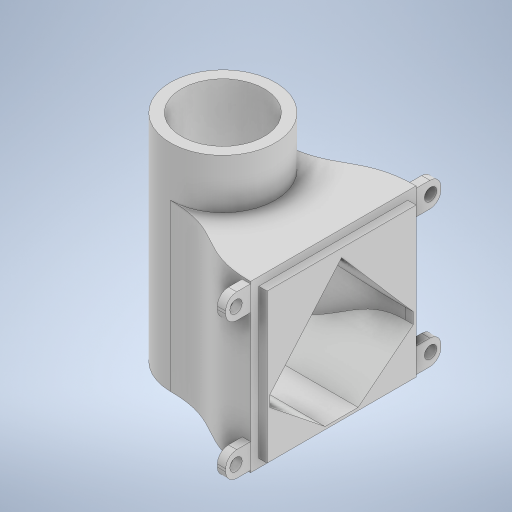
# Autodesk Inventor part: CO-1-01-eStopMountBottom
Saved by Autodesk Inventor 2024 (Build 280153000, 153)
## iProperties
Created: 2023-11-21
Part Number: CO-1-01-eStopMountBottom
Material: Generic
Document SubType Name: Modeling
Designer: t205b
Density: 1 g/cm^3
Appearance: Default
Author: t205b
Autodesk Inventor part; units mm, degrees
ref_plane "XZ Plane" through (0, 0, 0) normal (0, 1, 0) x (-1, 0, 0)
ref_plane "XY Plane" through (0, 0, 0) normal (0, 0, 1) x (1, 0, 0)
sketch "Sketch1" plane through (0, 0, 0) normal (0, 1, 0) x (-1, 0, 0)
  circle A0 centre (0, 0) radius 7.5
  circle A1 centre (0, 0) radius 9.5
  dimension "d0" = 19
  dimension "d1" = 2
  constraints: 2 centre point, 2 coincident
  measures "d0" diameter of A1
  measures "d1" radial gap between concentric circles of A0 A1
extrude "Extrusion1" add sketch "Sketch1" along normal blind 12
ref_plane "Work Plane1" through (9.5, 0, 0) normal (1, 0, 0) x (0, 1, 0)
sketch "Sketch2" plane through (9.5, 0, 0) normal (1, 0, 0) x (0, 1, 0)
  line L0 (-27, 15) -> (-27, -15)
  line L1 (-27, -15) -> (3, -15)
  line L2 (3, -15) -> (3, 15)
  line L3 (3, 15) -> (-27, 15)
  line L4 (-17, -13) -> (-15, -13)
  line L5 (-15, -13) -> (0, 0)
  line L6 (0, 0) -> (-15, 13)
  line L7 (-15, 13) -> (-17, 13)
  line L8 (0, 9.5) -> (12, 9.5) projected
  line L9 (0, -9.5) -> (12, -9.5) projected
  line L10 (0, -9.5) -> (0, 9.5) projected
  line L11 (-25, 3) -> (-25, -3)
  line L12 (-25, -3) -> (-17, -13)
  line L13 (-25, 3) -> (-17, 13)
  line L14 (-22.8, 0) -> (17.8, 0) projected
  line L15 (3, -10.2382) -> (-1.1045, -15)
  point P0 (0, 0)
  dimension "d5" = 30
  dimension "d6" = 2
  dimension "d7" = 2
  dimension "d9" = 26
  dimension "d10" = 13
  dimension "d11" = 3
  dimension "d12" = 3
  dimension "d13" = 30
  dimension "d17" = 2
  dimension "d18" = 2
  dimension "d20" = 2
  dimension "d21" = 6
  dimension "d22" = 3
  dimension "d53" = 15
  dimension "d97" = 8
  dimension "d98" = 8
  constraints: 24 end point, 2 perpendicular, 2 point on line, 2 vertical, 1 parallel
  measures "d5" distance between parallel lines of L1 L3
  measures "d6" distance between parallel lines of L3 L7
  measures "d7" distance between parallel lines of L1 L4
  measures "d9" distance between parallel lines of L7 L4
  measures "d10" distance from line of L5.end L4
  measures "d11" distance from line of L2 L5.end
  measures "d12" distance between parallel lines of L2 L10
  measures "d13" distance of L0.end L1.end
  measures "d17" distance of L4.start L4.end
  measures "d18" distance of L6.end L7.end
  measures "d20" distance between parallel lines of L11 L0
  measures "d21" distance of L11.start L11.end
  measures "d22" distance from line of L14 L11.end
  measures "d53" distance between parallel lines of L14 L1
  measures "d97" horizontal distance of L11.end L4.start
  measures "d98" horizontal distance of L11.start L7.end
extrude "Extrusion2" add sketch "Sketch2" along normal blind 12 and the other way blind 19
sketch "Sketch4" plane through (21.5, 0, 0) normal (1, 0, 0) x (0, 0, -1)
  circle A0 centre (-17.625, -24.375) radius 1.125
  circle A1 centre (-17.625, 0.375) radius 1.125
  circle A2 centre (17.625, -24.375) radius 1.125
  line L0 (7.5, 12) -> (7.5, 3) projected
  circle A3 centre (17.625, 0.375) radius 1.125
  line L1 (-15, 3) -> (-15, -27) projected
  line L2 (-15, -27) -> (15, -27) projected
  line L3 (15, -27) -> (15, 3) projected
  line L4 (15, 3) -> (-15, 3) projected
  line L5 (0, 0) -> (13, -15) projected
  line L6 (13, -15) -> (13, -17) projected
  line L7 (13, -17) -> (3, -25) projected
  line L8 (3, -25) -> (-3, -25) projected
  line L9 (-3, -25) -> (-13, -17) projected
  line L10 (-13, -17) -> (-13, -15) projected
  line L11 (-13, -15) -> (0, 0) projected
  line L12 (-13.5, -25.5) -> (-13.5, 1.5)
  line L13 (-13.5, 1.5) -> (13.5, 1.5)
  line L14 (13.5, 1.5) -> (13.5, -25.5)
  line L15 (13.5, -25.5) -> (-13.5, -25.5)
  point P0 (0, 0)
  dimension "d25" = 2.25
  dimension "d26" = 30
  dimension "d27" = 30
  dimension "d35" = 1.5
  dimension "d55" = 2.625
  dimension "d57" = 2.625
  dimension "d58" = 2.625
  dimension "d61" = 2.625
  dimension "d76" = 2.625
  dimension "d77" = 2.625
  dimension "d78" = 2.625
  dimension "d79" = 2.625
  constraints: 8 end point, 4 centre point, 3 equal radius, 3 other
  measures "d25" diameter of A0
  measures "d26" distance between parallel lines of L3 L1
  measures "d27" distance of L1.start L1.end
  measures "d35" distance between parallel lines of L1 L12
  measures "d55" distance from line of L4 A3.centre
  measures "d57" distance from line of L4 A1.centre
  measures "d58" distance from line of L2 A0.centre
  measures "d61" distance from line of L2 A2.centre
  measures "d76" distance from line of L3 A3.centre
  measures "d77" distance from line of L3 A2.centre
  measures "d78" distance from line of L1 A0.centre
  measures "d79" distance from line of L1 A1.centre
extrude "Extrusion4" cut sketch "Sketch4" against normal blind 1.5 contours L4 L3 L2 L1
sketch "Sketch8" plane through (0, 3, 0) normal (0, 1, 0) x (1, 0, 0)
  point P0 (0, 0)
  point P1 (0, 0)
  constraints: 1 coincident
hole "Hole2" at (0, 3, 0) direction (0, -1, 0) diameter 15 depth 10 tip angle 118
sketch "Sketch9" plane through (0, 3, 0) normal (0, 1, 0) x (1, 0, 0)
  line L0 (20, -15) -> (20, 15) projected
  line L1 (-9.5, 15) -> (20, 15) projected
  line L2 (-9.5, 0) -> (-9.5, 15) projected
  circle A0 centre (0, 0) radius 9.5 projected
  line L3 (-9.5, -15) -> (-9.5, 0) projected
  line L4 (20, -15) -> (-9.5, -15) projected
  line L5 (-9.5, 15) -> (20, 15) projected
  line L6 (0, 9.5) -> (10, 9.5) construction
  line L7 (10, 9.5) -> (10, 15) construction
  line L8 (10, 15) -> (20, 15) construction
  spline S0 degree 3 poles (0, 9.5) (10, 9.5) (10, 15) (20, 15) knots 1 1 1 1 2 2 2 2
  circle A1 centre (0, 0) radius 9.5 projected
  line L9 (-9.5, 15) -> (20, 15) projected
  line L10 (-15.7, 0) -> (27.7, 0) projected
  line L11 (0, -9.5) -> (10, -9.5) construction
  line L12 (10, -9.5) -> (10, -15) construction
  line L13 (10, -15) -> (20, -15) construction
  spline S1 degree 3 poles (0, -9.5) (10, -9.5) (10, -15) (20, -15) knots 1 1 1 1 2 2 2 2
  line L14 (20, -15) -> (20, -13)
  line L15 (-9.5, -15) -> (20, -15) projected
  circle A2 centre (0, 0) radius 7.5 projected
  line L16 (0, -9.5) -> (0, -7.5)
  line L17 (0, 9.5) -> (0, 7.5)
  line L18 (20, 15) -> (20, 13)
  spline S2 degree 5 poles (0, 7.5) (1.3329, 7.4998) (2.6642, 7.5767) (3.9935, 7.7452) (6.2499, 8.2593) (8.388, 9.1326) (9.262, 9.5613) (10.8348, 10.4267) (12.4076, 11.2917) (13.1436, 11.6655) (14.9046, 12.3988) (16.7696, 12.8147) (17.8461, 12.941) (18.922, 13.0004) (20, 13) knots 0 0 0 0 0 0 0.316871 0.316871 0.316871 0.547827 0.547827 0.547827 0.743764 0.743764 0.743764 1 1 1 1 1 1
  spline S3 degree 5 poles (0, -7.5) (1.3329, -7.4998) (2.6642, -7.5767) (3.9935, -7.7452) (6.2499, -8.2593) (8.388, -9.1326) (9.262, -9.5613) (10.8348, -10.4267) (12.4076, -11.2917) (13.1436, -11.6655) (14.9046, -12.3988) (16.7696, -12.8147) (17.8461, -12.941) (18.922, -13.0004) (20, -13) knots 0 0 0 0 0 0 0.316871 0.316871 0.316871 0.547827 0.547827 0.547827 0.743764 0.743764 0.743764 1 1 1 1 1 1
  point P0 (0, 0)
  point P1 (20, 15)
  point P2 (5.064, -8.0378)
  point P3 (5.064, 8.0378)
  dimension "d70" = 2
  dimension "d71" = 2
  dimension "d69" = 20
  constraints: 8 end point, 4 symmetric about line, 3 perpendicular, 2 collinear, 2 tangent, 1 horizontal, 1 parallel, 1 point on circle, 1 point on line, 1 vertical, 12 other
  measures "d69" horizontal distance of L8.end L6.start
extrude "Extrusion7" cut sketch "Sketch9" against normal through all contours L4 L3 A0 S1 | L2 L1 S0 A0
extrude "Extrusion8" add sketch "Sketch9" against normal blind 30 contours S1 A0 S3 L0 | L16 S3 A0 | A0 L10 A2 L16 | A0 L17 A2 L10 | S2 A0 S0 L0 | A0 S2 L17
sketch "Sketch11" plane through (20, 0, 0) normal (1, 0, 0) x (0, 0, -1)
  line L0 (-15, 2.625) -> (-19.5, 2.625)
  line L1 (-19.5, 2.625) -> (-19.5, -1.875)
  line L2 (-19.5, -1.875) -> (-15, -1.875)
  line L3 (-15, -22.125) -> (-19.5, -22.125)
  line L4 (-19.5, -22.125) -> (-19.5, -26.625)
  line L5 (-19.5, -26.625) -> (-15, -26.625)
  circle A0 centre (-17.625, 0.375) radius 1.125 projected
  line L6 (15, 3) -> (-15, 3) projected
  line L7 (0, -34.8003) -> (0, 19.8) projected
  line L8 (15, 2.625) -> (19.5, 2.625)
  line L9 (19.5, 2.625) -> (19.5, -1.875)
  line L10 (19.5, -1.875) -> (15, -1.875)
  line L11 (15, -22.125) -> (19.5, -22.125)
  line L12 (19.5, -22.125) -> (19.5, -26.625)
  line L13 (19.5, -26.625) -> (15, -26.625)
  line L14 (15, -27) -> (-15, -27) projected
  line L15 (-15, -27) -> (-15, 3) projected
  line L16 (13.5, -25.5) -> (13.5, 1.5) projected
  line L17 (15, 3) -> (15, -27) projected
  point P0 (0, 0)
  dimension "d80" = 4.5
  dimension "d82" = 4.5
  dimension "d92" = 0.375
  dimension "d93" = 2.25
  dimension "d94" = 4.5
  dimension "d95" = 4.5
  dimension "d96" = 0.375
  constraints: 24 end point, 8 symmetric about line, 4 perpendicular, 4 point on line, 2 horizontal
  measures "d80" distance of L0.end L1.end
  measures "d82" distance between parallel lines of L5 L3
  measures "d92" distance between parallel lines of L6 L0
  measures "d93" diameter of A0
  measures "d94" distance of L1.end L2.end
  measures "d95" distance of L4.end L5.end
  measures "d96" distance between parallel lines of L5 L14
extrude "Extrusion9" add sketch "Sketch11" against normal blind 1.5 contours L15 L2 L1 L0 | L15 L5 L4 L3 | L8 L9 L10 L17 | L17 L11 L12 L13
extrude "Extrusion3" cut sketch "Sketch4" against normal blind 6 contours A0 | A1 | A2 | A3
fillet "Fillet1" radius 2 8 edges at (19.25, 2.625, 19.5) (19.25, -1.875, 19.5) (19.25, -22.125, 19.5) (19.25, -26.625, 19.5) (19.25, -26.625, -19.5) (19.25, -22.125, -19.5) (19.25, 2.625, -19.5) (19.25, -1.875, -19.5)
equation "\"d7\" = d6"
equation "\"d10\" = 0.5 * d9"
equation "\"d18\" = d17"
equation "\"d21\" = d5 + 2 * d17 - 2 * d16 - 2 * d7"
equation "\"d22\" = 0.5 * d21"
equation "\"d53\" = 0.5 * d5"
equation "\"d98\" = d97"
equation "\"d55\" = d54"
equation "\"d57\" = d55"
equation "\"d58\" = d56"
equation "\"d61\" = d60"
equation "\"d77\" = d76"
equation "\"d78\" = d76"
equation "\"d79\" = d78"
equation "\"d82\" = d80"
equation "\"d94\" = d80"
equation "\"d95\" = d82"
equation "\"d56\" = d54"
equation "\"d60\" = d55"
equation "\"d16\" = 12"
equation "\"d54\" = 2.625"
body "Solid1"
